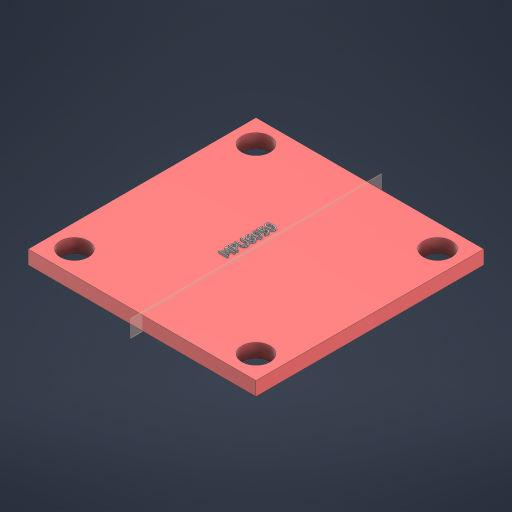
# Autodesk Inventor part: IMU Module
Saved by Autodesk Inventor 2023 (Build 270158000, 158)
## iProperties
Created: 2023-10-20
Part Number: IMU Module
Material: Generic
Document SubType Name: Modeling
Designer: nick_
Density: 1 g/cm^3
Appearance: Default
Author: nick_
Autodesk Inventor part; units mm, degrees
ref_plane "YZ Plane" through (0, 0, 0) normal (1, 0, 0) x (0, 1, 0)
ref_plane "XZ Plane" through (0, 0, 0) normal (0, 1, 0) x (-1, 0, 0)
ref_plane "XY Plane" through (0, 0, 0) normal (0, 0, 1) x (1, 0, 0)
sketch "Sketch1" plane through (0, 0, 0) normal (0, 1, 0) x (-1, 0, 0)
  line L0 (-12.6, 12.6) -> (12.6, 12.6)
  line L1 (12.6, 12.6) -> (12.6, -12.6)
  line L2 (12.6, -12.6) -> (-12.6, -12.6)
  line L3 (-12.6, -12.6) -> (-12.6, 12.6)
  line L4 (-12.6, 12.6) -> (12.6, -12.6) construction
  line L5 (12.6, 12.6) -> (-12.6, -12.6) construction
  point P0 (0, 0)
  dimension "d0" = 25.2
  dimension "d1" = 25.2
  constraints: 12 end point, 2 midpoint, 2 parallel, 1 horizontal, 1 perpendicular
  measures "d0" distance of L1.end L2.end
  measures "d1" distance of L0.end L1.end
extrude "Extrusion1" add sketch "Sketch1" along normal blind 1.53
sketch "Sketch2" plane through (0, 1.53, 0) normal (0, 1, 0) x (1, 0, 0)
  line L0 (12.6, -12.6) -> (12.6, 12.6) projected
  line L1 (12.6, 12.6) -> (-12.6, 12.6) projected
  line L2 (-12.6, 12.6) -> (-12.6, -12.6) projected
  line L3 (-12.6, -12.6) -> (12.6, -12.6) projected
  point P0 (0, 0)
  point P1 (10.05, 10.05)
  point P2 (-10.05, 10.05)
  point P3 (-10.05, -10.05)
  point P4 (10.05, -10.05)
  dimension "d4" = 2.55
  dimension "d5" = 2.55
  dimension "d30" = 2.55
  dimension "d31" = 2.55
  constraints: 2 horizontal alignment, 2 vertical alignment
  measures "d4" distance from line of L0 point (10.05, 10.05)
  measures "d5" distance from line of L1 point (10.05, 10.05)
  measures "d30" distance from line of L2 point (-10.05, 10.05)
  measures "d31" distance from line of L3 point (10.05, -10.05)
hole "Hole1" at (10.05, 1.53, -10.05) at (-10.05, 1.53, -10.05) at (10.05, 1.53, 10.05) at (-10.05, 1.53, 10.05) direction (0, -1, 0) diameter 3.1 end through all
sketch "Sketch6" plane through (0, 1.53, 0) normal (0, 1, 0) x (1, 0, 0)
  line L0 (-1.7084, -23.5263) -> (-1.7084, 24.1475) construction
  line L1 (-1.7084, 24.1475) -> (7.2695, 24.1475) construction
  line L2 (7.2695, 24.1475) -> (7.2695, -23.5263) construction
  line L3 (7.2695, -23.5263) -> (-1.7084, -23.5263) construction
  line L4 (-0.6882, -1.5917) -> (-0.6882, -1.7246)
  line L5 (-0.6882, -1.7246) -> (-1.5496, -1.7246)
  line L6 (-1.5496, -1.7246) -> (-0.9637, -1.9856)
  line L7 (-0.9637, -1.9856) -> (-0.9637, -2.0666)
  line L8 (-0.9637, -2.0666) -> (-1.5496, -2.3251)
  line L9 (-1.5496, -2.3251) -> (-0.6882, -2.3251)
  line L10 (-0.6882, -2.3251) -> (-0.6882, -2.4491)
  line L11 (-0.6882, -2.4491) -> (-1.6882, -2.4491)
  line L12 (-1.6882, -2.4491) -> (-1.6882, -2.2676)
  line L13 (-1.6882, -2.2676) -> (-1.1314, -2.018)
  line L14 (-1.1314, -2.018) -> (-1.6882, -1.7765)
  line L15 (-1.6882, -1.7765) -> (-1.6882, -1.5917)
  line L16 (-1.6882, -1.5917) -> (-0.6882, -1.5917)
  spline S0 degree 2 poles (-1.3867, -0.757) (-1.3219, -0.757) (-1.2052, -0.8032) (-1.1647, -0.8446) knots 0 0 0 1 2 2 2
  spline S1 degree 2 poles (-1.1647, -0.8446) (-1.1136, -0.8964) (-1.0609, -1.0366) (-1.0609, -1.1436) knots 0 0 0 1 2 2 2
  line L17 (-1.0609, -1.1436) -> (-1.0609, -1.2562)
  line L18 (-1.0609, -1.2562) -> (-0.6882, -1.2562)
  line L19 (-0.6882, -1.2562) -> (-0.6882, -1.3891)
  line L20 (-0.6882, -1.3891) -> (-1.6882, -1.3891)
  line L21 (-1.6882, -1.3891) -> (-1.6882, -1.1379)
  spline S2 degree 2 poles (-1.6882, -1.1379) (-1.6882, -1.0488) (-1.659, -0.924) (-1.6258, -0.8762) knots 0 0 0 1 2 2 2
  spline S3 degree 2 poles (-1.6258, -0.8762) (-1.5877, -0.8203) (-1.4702, -0.757) (-1.3867, -0.757) knots 0 0 0 1 2 2 2
  spline S4 degree 2 poles (-1.3827, -0.8956) (-1.4345, -0.8956) (-1.5107, -0.9313) (-1.535, -0.9677) knots 0 0 0 1 2 2 2
  spline S5 degree 2 poles (-1.535, -0.9677) (-1.5561, -0.9993) (-1.5731, -1.0836) (-1.5731, -1.146) knots 0 0 0 1 2 2 2
  line L22 (-1.5731, -1.146) -> (-1.5731, -1.2562)
  line L23 (-1.5731, -1.2562) -> (-1.1744, -1.2562)
  line L24 (-1.1744, -1.2562) -> (-1.1744, -1.1655)
  spline S6 degree 2 poles (-1.1744, -1.1655) (-1.1744, -1.0844) (-1.2003, -0.9848) (-1.2344, -0.9523) knots 0 0 0 1 2 2 2
  spline S7 degree 2 poles (-1.2344, -0.9523) (-1.2643, -0.9224) (-1.3348, -0.8956) (-1.3827, -0.8956) knots 0 0 0 1 2 2 2
  spline S8 degree 2 poles (-0.6671, -0.2814) (-0.6671, -0.3697) (-0.7133, -0.501) (-0.7595, -0.5472) knots 0 0 0 1 2 2 2
  spline S9 degree 2 poles (-0.7595, -0.5472) (-0.8113, -0.5998) (-0.9572, -0.6428) (-1.0642, -0.6428) knots 0 0 0 1 2 2 2
  line L25 (-1.0642, -0.6428) -> (-1.6882, -0.6428)
  line L26 (-1.6882, -0.6428) -> (-1.6882, -0.5099)
  line L27 (-1.6882, -0.5099) -> (-1.0642, -0.5099)
  spline S10 degree 2 poles (-1.0642, -0.5099) (-0.9945, -0.5099) (-0.9005, -0.4921) (-0.8624, -0.4669) knots 0 0 0 1 2 2 2
  spline S11 degree 2 poles (-0.8624, -0.4669) (-0.8219, -0.4402) (-0.7805, -0.3478) (-0.7805, -0.2814) knots 0 0 0 1 2 2 2
  spline S12 degree 2 poles (-0.7805, -0.2814) (-0.7805, -0.219) (-0.8219, -0.1217) (-0.8624, -0.095) knots 0 0 0 1 2 2 2
  spline S13 degree 2 poles (-0.8624, -0.095) (-0.9005, -0.0698) (-0.9937, -0.052) (-1.0609, -0.052) knots 0 0 0 1 2 2 2
  line L28 (-1.0609, -0.052) -> (-1.6882, -0.052)
  line L29 (-1.6882, -0.052) -> (-1.6882, 0.0809)
  line L30 (-1.6882, 0.0809) -> (-1.0642, 0.0809)
  spline S14 degree 2 poles (-1.0642, 0.0809) (-0.9596, 0.0809) (-0.8105, 0.0387) (-0.7595, -0.0147) knots 0 0 0 1 2 2 2
  spline S15 degree 2 poles (-0.7595, -0.0147) (-0.7125, -0.0626) (-0.6671, -0.189) (-0.6671, -0.2814) knots 0 0 0 1 2 2 2
  spline S16 degree 2 poles (-1.0123, 0.875) (-0.9353, 0.875) (-0.8049, 0.824) (-0.7611, 0.781) knots 0 0 0 1 2 2 2
  spline S17 degree 2 poles (-0.7611, 0.781) (-0.7149, 0.7365) (-0.6671, 0.6246) (-0.6671, 0.5574) knots 0 0 0 1 2 2 2
  spline S18 degree 2 poles (-0.6671, 0.5574) (-0.6671, 0.4901) (-0.7125, 0.3791) (-0.7579, 0.337) knots 0 0 0 1 2 2 2
  spline S19 degree 2 poles (-0.7579, 0.337) (-0.8122, 0.2851) (-0.9945, 0.2267) (-1.1274, 0.2267) knots 0 0 0 1 2 2 2
  spline S20 degree 2 poles (-1.1274, 0.2267) (-1.2579, 0.2267) (-1.4677, 0.2802) (-1.5455, 0.3361) knots 0 0 0 1 2 2 2
  spline S21 degree 2 poles (-1.5455, 0.3361) (-1.6217, 0.3904) (-1.7068, 0.5622) (-1.7068, 0.6749) knots 0 0 0 1 2 2 2
  spline S22 degree 2 poles (-1.7068, 0.6749) (-1.7068, 0.7081) (-1.7003, 0.7665) (-1.693, 0.7883) knots 0 0 0 1 2 2 2
  line L31 (-1.693, 0.7883) -> (-1.5642, 0.7883)
  line L32 (-1.5642, 0.7883) -> (-1.5642, 0.7827)
  spline S23 degree 2 poles (-1.5642, 0.7827) (-1.5739, 0.764) (-1.5909, 0.696) (-1.5909, 0.6571) knots 0 0 0 1 2 2 2
  spline S24 degree 2 poles (-1.5909, 0.6571) (-1.5909, 0.5323) (-1.4224, 0.3791) (-1.257, 0.3645) knots 0 0 0 1 2 2 2
  spline S25 degree 2 poles (-1.257, 0.3645) (-1.2903, 0.4123) (-1.3267, 0.5128) (-1.3267, 0.5728) knots 0 0 0 1 2 2 2
  spline S26 degree 2 poles (-1.3267, 0.5728) (-1.3267, 0.6311) (-1.3032, 0.7186) (-1.2676, 0.7665) knots 0 0 0 1 2 2 2
  spline S27 degree 2 poles (-1.2676, 0.7665) (-1.2263, 0.8216) (-1.0982, 0.875) (-1.0123, 0.875) knots 0 0 0 1 2 2 2
  spline S28 degree 2 poles (-1.0066, 0.7389) (-1.0682, 0.7389) (-1.1517, 0.7065) (-1.1809, 0.6708) knots 0 0 0 1 2 2 2
  spline S29 degree 2 poles (-1.1809, 0.6708) (-1.2019, 0.6441) (-1.2157, 0.5776) (-1.2157, 0.5428) knots 0 0 0 1 2 2 2
  spline S30 degree 2 poles (-1.2157, 0.5428) (-1.2157, 0.4958) (-1.1874, 0.4075) (-1.1606, 0.3645) knots 0 0 0 1 2 2 2
  spline S31 degree 2 poles (-1.1606, 0.3645) (-1.146, 0.3637) (-1.1185, 0.3621) (-1.0974, 0.3621) knots 0 0 0 1 2 2 2
  spline S32 degree 2 poles (-1.0974, 0.3621) (-0.9937, 0.3621) (-0.8664, 0.4026) (-0.8332, 0.4334) knots 0 0 0 1 2 2 2
  spline S33 degree 2 poles (-0.8332, 0.4334) (-0.8016, 0.4618) (-0.7765, 0.5233) (-0.7765, 0.5582) knots 0 0 0 1 2 2 2
  spline S34 degree 2 poles (-0.7765, 0.5582) (-0.7765, 0.6392) (-0.8916, 0.7389) (-1.0066, 0.7389) knots 0 0 0 1 2 2 2
  spline S35 degree 2 poles (-1.1882, 1.6157) (-0.9191, 1.6157) (-0.6671, 1.4593) (-0.6671, 1.2964) knots 0 0 0 1 2 2 2
  spline S36 degree 2 poles (-0.6671, 1.2964) (-0.6671, 1.1311) (-0.924, 0.9763) (-1.1874, 0.9763) knots 0 0 0 1 2 2 2
  spline S37 degree 2 poles (-1.1874, 0.9763) (-1.458, 0.9763) (-1.7084, 1.1327) (-1.7084, 1.2964) knots 0 0 0 1 2 2 2
  spline S38 degree 2 poles (-1.7084, 1.2964) (-1.7084, 1.4609) (-1.4491, 1.6157) (-1.1882, 1.6157) knots 0 0 0 1 2 2 2
  spline S39 degree 2 poles (-0.8835, 1.4439) (-0.9329, 1.4634) (-1.0852, 1.4796) (-1.1882, 1.4796) knots 0 0 0 1 2 2 2
  spline S40 degree 2 poles (-1.1882, 1.4796) (-1.2911, 1.4796) (-1.4426, 1.4634) (-1.4937, 1.4431) knots 0 0 0 1 2 2 2
  spline S41 degree 2 poles (-1.4937, 1.4431) (-1.5447, 1.4229) (-1.5974, 1.3524) (-1.5974, 1.2964) knots 0 0 0 1 2 2 2
  spline S42 degree 2 poles (-1.5974, 1.2964) (-1.5974, 1.2405) (-1.5447, 1.1684) (-1.4921, 1.1473) knots 0 0 0 1 2 2 2
  spline S43 degree 2 poles (-1.4921, 1.1473) (-1.441, 1.1271) (-1.2854, 1.1125) (-1.1874, 1.1125) knots 0 0 0 1 2 2 2
  spline S44 degree 2 poles (-1.1874, 1.1125) (-1.082, 1.1125) (-0.941, 1.1255) (-0.8859, 1.1465) knots 0 0 0 1 2 2 2
  spline S45 degree 2 poles (-0.8859, 1.1465) (-0.834, 1.166) (-0.7781, 1.2381) (-0.7781, 1.2964) knots 0 0 0 1 2 2 2
  spline S46 degree 2 poles (-0.7781, 1.2964) (-0.7781, 1.3515) (-0.8308, 1.4237) (-0.8835, 1.4439) knots 0 0 0 1 2 2 2
  spline S47 degree 2 poles (-1.0058, 2.3499) (-0.9337, 2.3499) (-0.8105, 2.3037) (-0.7652, 2.2616) knots 0 0 0 1 2 2 2
  spline S48 degree 2 poles (-0.7652, 2.2616) (-0.7198, 2.2195) (-0.6671, 2.0938) (-0.6671, 2.0161) knots 0 0 0 1 2 2 2
  spline S49 degree 2 poles (-0.6671, 2.0161) (-0.6671, 1.9447) (-0.6987, 1.8054) (-0.7238, 1.7543) knots 0 0 0 1 2 2 2
  line L33 (-0.7238, 1.7543) -> (-0.8656, 1.7543)
  line L34 (-0.8656, 1.7543) -> (-0.8656, 1.764)
  spline S50 degree 2 poles (-0.8656, 1.764) (-0.8543, 1.7794) (-0.8251, 1.837) (-0.8122, 1.8718) knots 0 0 0 1 2 2 2
  spline S51 degree 2 poles (-0.8122, 1.8718) (-0.7984, 1.9115) (-0.783, 1.9772) (-0.783, 2.0185) knots 0 0 0 1 2 2 2
  spline S52 degree 2 poles (-0.783, 2.0185) (-0.783, 2.059) (-0.8122, 2.1352) (-0.8438, 2.1627) knots 0 0 0 1 2 2 2
  spline S53 degree 2 poles (-0.8438, 2.1627) (-0.8737, 2.1879) (-0.9532, 2.2138) (-1.0066, 2.2138) knots 0 0 0 1 2 2 2
  spline S54 degree 2 poles (-1.0066, 2.2138) (-1.0601, 2.2138) (-1.1282, 2.1846) (-1.1509, 2.1571) knots 0 0 0 1 2 2 2
  spline S55 degree 2 poles (-1.1509, 2.1571) (-1.176, 2.1287) (-1.1971, 2.0444) (-1.1971, 1.9934) knots 0 0 0 1 2 2 2
  spline S56 degree 2 poles (-1.1971, 1.9934) (-1.1971, 1.9383) (-1.1801, 1.8289) (-1.1728, 1.7956) knots 0 0 0 1 2 2 2
  line L35 (-1.1728, 1.7956) -> (-1.6882, 1.7956)
  line L36 (-1.6882, 1.7956) -> (-1.6882, 2.3443)
  line L37 (-1.6882, 2.3443) -> (-1.5707, 2.3443)
  line L38 (-1.5707, 2.3443) -> (-1.5707, 1.9245)
  line L39 (-1.5707, 1.9245) -> (-1.304, 1.9245)
  spline S57 degree 2 poles (-1.304, 1.9245) (-1.3073, 1.9488) (-1.3097, 1.9958) (-1.3097, 2.0152) knots 0 0 0 1 2 2 2
  spline S58 degree 2 poles (-1.3097, 2.0152) (-1.3097, 2.0922) (-1.2846, 2.1984) (-1.2473, 2.247) knots 0 0 0 1 2 2 2
  spline S59 degree 2 poles (-1.2473, 2.247) (-1.21, 2.2964) (-1.0966, 2.3499) (-1.0058, 2.3499) knots 0 0 0 1 2 2 2
  spline S60 degree 2 poles (-1.1882, 3.1165) (-0.9191, 3.1165) (-0.6671, 2.9601) (-0.6671, 2.7973) knots 0 0 0 1 2 2 2
  spline S61 degree 2 poles (-0.6671, 2.7973) (-0.6671, 2.6319) (-0.924, 2.4772) (-1.1874, 2.4772) knots 0 0 0 1 2 2 2
  spline S62 degree 2 poles (-1.1874, 2.4772) (-1.458, 2.4772) (-1.7084, 2.6336) (-1.7084, 2.7973) knots 0 0 0 1 2 2 2
  spline S63 degree 2 poles (-1.7084, 2.7973) (-1.7084, 2.9618) (-1.4491, 3.1165) (-1.1882, 3.1165) knots 0 0 0 1 2 2 2
  spline S64 degree 2 poles (-0.8835, 2.9447) (-0.9329, 2.9642) (-1.0852, 2.9804) (-1.1882, 2.9804) knots 0 0 0 1 2 2 2
  spline S65 degree 2 poles (-1.1882, 2.9804) (-1.2911, 2.9804) (-1.4426, 2.9642) (-1.4937, 2.9439) knots 0 0 0 1 2 2 2
  spline S66 degree 2 poles (-1.4937, 2.9439) (-1.5447, 2.9237) (-1.5974, 2.8532) (-1.5974, 2.7973) knots 0 0 0 1 2 2 2
  spline S67 degree 2 poles (-1.5974, 2.7973) (-1.5974, 2.7413) (-1.5447, 2.6692) (-1.4921, 2.6481) knots 0 0 0 1 2 2 2
  spline S68 degree 2 poles (-1.4921, 2.6481) (-1.441, 2.6279) (-1.2854, 2.6133) (-1.1874, 2.6133) knots 0 0 0 1 2 2 2
  spline S69 degree 2 poles (-1.1874, 2.6133) (-1.082, 2.6133) (-0.941, 2.6263) (-0.8859, 2.6473) knots 0 0 0 1 2 2 2
  spline S70 degree 2 poles (-0.8859, 2.6473) (-0.834, 2.6668) (-0.7781, 2.7389) (-0.7781, 2.7973) knots 0 0 0 1 2 2 2
  spline S71 degree 2 poles (-0.7781, 2.7973) (-0.7781, 2.8524) (-0.8308, 2.9245) (-0.8835, 2.9447) knots 0 0 0 1 2 2 2
  point P0 (0, 0)
  dimension "d0" = 25.2
  dimension "d1" = 25.2
  constraints: 2 other
emboss "Emboss1" sketch "Sketch6" operation add depth 0.2 direction (0, -1, 0)
ref_plane "Work Plane1" through (0, 0, 12.6) normal (1, 0, 0) x (0, 0, -1)
equation "\"d5\" = d4"
equation "\"d30\" = d4"
equation "\"d31\" = d4"
body "Solid1"
